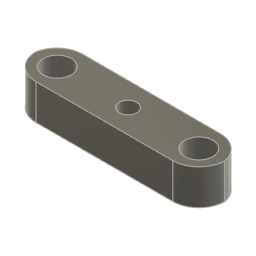
_V2 RealSense Mount.c3c66d58-4b16-4023-b535-7b466959c17c (Autodesk Fusion 360 design; units mm, degrees)
Autodesk Fusion 360 part; units mm, degrees
note: some values were not read from the file. Set by a fixed rule: which sketch regions a step uses.
sketch "Sketch1" plane through (0, 0, 0) normal (0, 1, 0) x (1, 0, 0)
  line L0 (0, 0) -> (20, 0)
  line L1 (20, 0) -> (20, -10)
  line L2 (20, -10) -> (0, -10)
  circle A0 centre (15, -5) radius 3
  circle A1 centre (15, -5) radius 1.9
  circle A2 centre (0, -5) radius 3
  circle A3 centre (0, -5) radius 1.9
  line L3 (0, -5) -> (0, -10)
  line L4 (15, -5) -> (15, -10)
  line L5 (20, -10) -> (20, -5)
  line L6 (0, 0) -> (0, -10)
  line L7 (12, -10) -> (12, -5)
  dimension "d2" = 5
  dimension "d3" = 3.8
  dimension "d4" = 6
  dimension "d5" = 10
  dimension "d19" = 15
  dimension "d20" = 12
  constraint coincident L0.start L6.start
  constraint horizontal L0
  constraint perpendicular L0 L1
  constraint perpendicular L1 L2
  constraint concentric A0 A1
  constraint concentric A2 A3
  constraint coincident A2.centre A3.centre
  constraint coincident L2 L3.end
  constraint perpendicular L2 L3
  constraint coincident A0.centre A1.centre
  constraint coincident L2 L4.end
  constraint perpendicular L2 L4
  constraint midpoint L1 L5.end
  constraint equal L4 L5
  constraint equal L3 L4
  constraint equal A1 A3
  constraint equal A0 A2
  constraint perpendicular L2 L6
  constraint midpoint A2.centre L6
  constraint coincident L2 L7.start
  constraint coincident A0 L7.end
  constraint tangent A0 L7
  constraint perpendicular L2 L7
  measures "d2" distance of L1 A0.centre
  measures "d3" diameter of A1
  measures "d4" diameter of A0
  measures "d5" distance of L0.end L1.end
  measures "d19" distance of A0.centre A2.centre
  measures "d20" distance of A2.centre L7
extrude "Extrude1" add sketch "Sketch1" along normal blind 7.5 contours L0 L1 L2 A0 A2 L3 L4 L5 L6 L7 | L2 A0 L4 L7
extrude "Extrude2" add sketch "Sketch1" along normal blind 3 contours A0
extrude "Extrude3" add sketch "Sketch1" along normal blind 7.5 and the other way blind -3.5 contours A2 A3 L3 L6 picked at (2.0756, -6.6102)
mirror "Mirror1" about plane through (0, 3.5, 6.9) normal (-1, 0, 0) of bodies 1 merged
fillet "Fillet1" radius 5.5 4 edges at (-20, 3.75, 10) (-20, 3.75, 0) (20, 3.75, 10) (20, 3.75, 0)
equation "d13 = -7.5 mm + 4 mm"
named bodies: "realsense mount"
